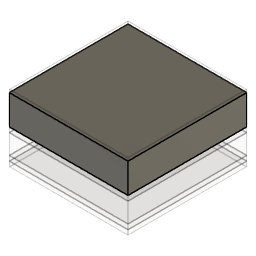
modele_fusion_V1.2 (Autodesk Fusion 360 design; units mm, degrees)
part number: 2026-06-02-09-50-29-074
part number: 2026-06-02-09-51-34-644
part number: 2026-06-02-10-02-59-264
part number: 2026-06-02-10-04-26-838
part number: 2026-06-02-16-27-04-294
part number: 2026-06-02-16-29-52-407
Autodesk Fusion 360 part; units mm, degrees
sketch "Esquisse1" plane through (0, 0, 0) normal (0, 0, 1) x (1, 0, 0) in component "Support"
sketch "Esquisse1 (2)" plane through (0, 0, 5) normal (0, 0, 1) x (-1, 0, 0) in component "Conducteur_haut"
sketch "Esquisse2" plane through (0, 0, 0) normal (0, 0, 1) x (1, 0, 0)
  line L0 (0, 0) -> (24, 0)
  line L1 (24, 0) -> (24, 20)
  line L2 (24, 20) -> (0, 20)
  line L3 (0, 20) -> (0, 0)
  dimension "d36" = 24
  dimension "d37" = 20
  constraint horizontal L0
  constraint vertical L1
  constraint horizontal L2
  constraint vertical L3
  constraint coincident L0.start L3.end
  measures "d36" distance of L0.start L0.end
  measures "d37" distance of L0.start L2.end
combine "Combiner1" [no effect]
sketch "Esquisse1 (3)" plane through (0, 0, 0) normal (0, 1, 0) x (1, 0, 0) in component "Mousse"
sketch "Esquisse2 (2)" plane through (0, 0, 12) normal (0, 0, 1) x (-1, 0, 0) in component "Mousse"
  line L0 (0, -20) -> (0, 0)
  line L1 (0, 0) -> (-24, 0)
  line L2 (-24, 0) -> (-24, -20)
  line L3 (-24, -20) -> (0, -20)
  line L4 (0, 0) -> (-24, 0)
  line L5 (-24, 0) -> (-24, -20)
  line L6 (-24, -20) -> (0, -20)
  line L7 (0, -20) -> (0, 0)
  dimension "d40" = 24
  dimension "d41" = 20
  constraint horizontal L4
  constraint vertical L5
  constraint horizontal L6
  constraint vertical L7
  constraint coincident L0.end L1.start
  measures "d40" distance of L0.end L1.end
  measures "d41" distance of L0.end L0.start
sketch "Esquisse3" plane through (0, 0, 0) normal (0, 0, 1) x (1, 0, 0)
  line L0 (0, 0) -> (24, 0)
  line L1 (24, 0) -> (24, 24)
  line L2 (24, 24) -> (0, 24)
  line L3 (0, 24) -> (0, 0)
  dimension "d44" = 24
  dimension "d45" = 24
  constraint horizontal L0
  constraint vertical L1
  constraint horizontal L2
  constraint vertical L3
  constraint coincident L0.start L3.end
  measures "d44" distance of L0.start L0.end
  measures "d45" distance of L0.start L2.end
extrude "Extrusion3" add sketch "Esquisse3" along normal blind 1 makes body 1
copy_body "CutPasteBodies3" bodies 1 removing the originals makes body 2 in component "Support"
extrude "Extrusion2" add 1 faces at (16, 8, 1) along direction (0, 0, 1) blind 1 separate body on bodies 2 makes body 3 in component "Conducteur_bas"
extrude "Extrusion4" add 1 faces at (16, 8, 2) along direction (0, 0, 1) blind 4 separate body on bodies 3 makes body 4 in component "Support"
extrude "Extrusion2'" add 1 faces at (16, 8, 6) along direction (0, 0, 1) blind 1 separate body on bodies 4 makes body 5 in component "Conducteur_haut"
extrude "Extrusion1" add 1 faces at (16, 8, 7) along direction (0, 0, 1) blind 6 separate body on bodies 5 makes body 6 in component "Mousse"
extrude "Extrusion2''" add 1 faces at (16, 8, 13) along direction (0, 0, 1) blind 0.6 separate body on bodies 6 makes body 7 in component "Plateau"
component "Support" placed x (1, 0, 0) y (0, 1, 0) z (0, 0, 1) at (0, 0, 0)
component "Conducteur_bas" placed x (1, 0, 0) y (0, 1, 0) z (0, 0, 1) at (0, 0, 0)
component "Conducteur_haut" placed x (1, 0, 0) y (0, 1, 0) z (0, 0, 1) at (0, 0, 0)
component "Mousse" placed x (1, 0, 0) y (0, 1, 0) z (0, 0, 1) at (0, 0, 0)
component "Plateau" placed x (1, 0, 0) y (0, 1, 0) z (0, 0, 1) at (0, 0, 0)
component "(Non enregistré)" placed x (1, 0, 0) y (0, 1, 0) z (0, 0, 1) at (0, 0, 0) in component "Conducteur_bas"
equation "Deltax = 8 mm"
equation "largeur_electrode = 8 mm"
equation "Longeur = 20 mm"
equation "d = 6 mm"
equation "Hauteur_support = 1 mm"
equation "deltad = 4 mm"
equation "Hauteur = d + Epaisseur_electrode + deltad + Hauteur_support"
equation "Largeur = Deltax + 2 * largeur_electrode"
equation "Epaisseur_electrode = 1 mm"
equation "Epaisseur_plateau = 0.6 mm"
equation "d36 = Largeur"
equation "d37 = Longeur"
equation "d40 = Largeur"
equation "d41 = Longeur"
equation "d44 = Largeur"
equation "d45 = Largeur"
equation "d46 = Hauteur_support"
equation "d48 = Epaisseur_electrode"
equation "d50 = deltad"
equation "d52 = Epaisseur_electrode"
equation "d54 = d"
equation "d56 = Epaisseur_plateau"
